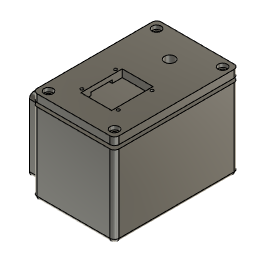
memento-mori (Autodesk Fusion 360 design; units mm, degrees)
Autodesk Fusion 360 part; units mm, degrees
sketch "pcb" plane through (0, 0, 0) normal (0, 0, 1) x (1, 0, 0)
  line L0 (0, 0) -> (40, 0)
  line L1 (40, 0) -> (40, 60.5)
  line L2 (40, 60.5) -> (0, 60.5)
  line L3 (0, 60.5) -> (0, 0)
  line L4 (2.25, 60.5) -> (2.25, 67.8)
  line L5 (2.25, 67.8) -> (21.25, 67.8)
  line L6 (21.25, 67.8) -> (21.25, 60.5)
  circle A0 centre (37.1, 57.8) radius 0.9
  line L7 (20, 0) -> (20, 60.5) construction
  line L8 (0, 30.25) -> (40, 30.25) construction
  circle A1 centre (2.9, 57.8) radius 0.9
  circle A2 centre (2.9, 2.7) radius 0.9
  circle A3 centre (37.1, 2.7) radius 0.9
  dimension "d1" = 40
  dimension "d2" = 60.5
  dimension "d5" = 2.25
  dimension "d6" = 19
  dimension "d7" = 7.3
  dimension "d12" = 1.8
  dimension "d13" = 1.8
  dimension "d14" = 2
  constraint horizontal L0
  constraint vertical L1
  constraint horizontal L2
  constraint vertical L3
  constraint coincident L0.start L3.end
  constraint coincident L2 L4.start
  constraint perpendicular L2 L4
  constraint perpendicular L4 L5
  constraint coincident L2 L6.end
  constraint perpendicular L2 L6
  constraint midpoint L0 L7.start
  constraint midpoint L2 L7.end
  constraint midpoint L3 L8.start
  constraint midpoint L1 L8.end
  constraint symmetric A0 L7 A1
  constraint symmetric A0 L8 A3
  constraint symmetric L8 A1 A2
  measures "d1" distance of L0.start L0.end
  measures "d2" distance of L0.start L2.end
  measures "d5" distance of L3 L4
  measures "d6" distance of L4.end L5.end
  measures "d7" distance of L5.end L6.end
  measures "d12" diameter of A0
  measures "d13" distance of L2 A0
  measures "d14" distance of L1 A0
extrude "Extrude1" add sketch "pcb" along normal blind 20 makes body 1
sketch "case" plane through (0, 0, 20) normal (0, 0, 1) x (-1, 0, 0)
  line L0 (-2.25, -60.5) -> (0, -60.5)
  line L1 (0, -60.5) -> (0, 0)
  line L2 (0, 0) -> (-40, 0)
  line L3 (-40, 0) -> (-40, -60.5)
  line L4 (-40, -60.5) -> (-21.25, -60.5)
  line L5 (-21.25, -60.5) -> (-21.25, -67.8)
  line L6 (-21.25, -67.8) -> (-2.25, -67.8)
  line L7 (-2.25, -67.8) -> (-2.25, -60.5)
  line L8 (7, -69.8) -> (-47, -69.8)
  line L9 (-47, -69.8) -> (-47, 12)
  line L10 (-47, 12) -> (7, 12)
  line L11 (7, 12) -> (7, -69.8)
  line L12 (-40, 0) -> (-40, -60.5)
  line L13 (0, -60.5) -> (0, 0)
  line L14 (0, 0) -> (-40, 0)
  line L15 (-2.25, -67.8) -> (-21.25, -67.8)
  circle A0 centre (-37.1, -2.7) radius 0.9
  circle A1 centre (-2.9, -2.7) radius 0.9
  circle A2 centre (-2.9, -57.8) radius 0.9
  circle A3 centre (-37.1, -57.8) radius 0.9
  line L16 (-44.25, 9.25) -> (4.25, 9.25)
  line L17 (4.25, 9.25) -> (4.25, -67.05)
  line L18 (4.25, -67.05) -> (-44.25, -67.05)
  line L19 (-44.25, -67.05) -> (-44.25, 9.25)
  dimension "d8" = 7
  dimension "d9" = 7
  dimension "d10" = 12
  dimension "d11" = 2
  dimension "d15" = 2.75
  constraint horizontal L8
  constraint vertical L9
  constraint horizontal L10
  constraint vertical L11
  measures "d8" distance of L9 L12
  measures "d9" distance of L11 L13
  measures "d10" distance of L10 L14
  measures "d11" distance of L8 L15
extrude "Extrude3" add sketch "case" against normal blind 8.5 from surface at -20 separate body contours L0 L1 L2 L3 L4 L5 L7 L12 L13 L14 L18 | L0 L1 L2 L3 L4 L5 L7 L12 L13 L14 L16 L17 L18 L19 | L5 L6 L7 L15 L18 | L8 L9 L10 L11 | A0 | A1 | A2 | A3 makes body 2
extrude "Extrude4" add sketch "case" along normal blind 45 from surface at -20 contours L5 L6 L7 L15 L18 | L8 L9 L10 L11 bodies 2
sketch "charge-panel" plane through (0, 69.8, 0) normal (0, 1, 0) x (-1, 0, 0)
  line L0 (-47, 45) -> (-47, -8.5)
  line L1 (-47, -8.5) -> (7, -8.5)
  line L2 (7, -8.5) -> (7, 45)
  line L3 (7, 45) -> (-47, 45)
  line L4 (-21.25, 0) -> (-21.25, 20)
  line L5 (-21.25, 20) -> (-2.25, 20) construction
  line L6 (-2.25, 0) -> (-2.25, 20)
  line L7 (-2.25, 0) -> (-21.25, 0)
  line L8 (-40, 20) -> (-21.25, 20)
  line L9 (-40, 0) -> (-40, 20)
  line L10 (-40, 0) -> (-21.25, 0)
  line L11 (0, 0) -> (0, 20)
  line L12 (-2.25, 0) -> (0, 0)
  line L13 (-2.25, 20) -> (0, 20)
  line L14 (-21.25, 25) -> (-2.25, 25)
  line L15 (-21.25, 25) -> (-26, 25)
  line L16 (-26, 25) -> (-26, 0)
  line L17 (-38, 25) -> (-34, 25)
  line L18 (-34, 25) -> (-34, 16.35)
  line L19 (-34, 16.35) -> (-38, 16.35)
  line L20 (-38, 16.35) -> (-38, 25)
  line L21 (-21.25, 10) -> (-2.25, 10)
  line L22 (-21.25, 20) -> (-21.25, 25)
  line L23 (-2.25, 25) -> (-2.25, 20)
  dimension "d28" = 4.75
  dimension "d29" = 8.65
  dimension "d30" = 4
  dimension "d32" = 2
  dimension "d160" = 10
  dimension "d161" = 15
  constraint coincident L4 L14.start
  constraint coincident L6 L14.end
  constraint perpendicular L6 L14
  constraint perpendicular L4 L15
  constraint coincident L10 L16.end
  constraint horizontal L17
  constraint vertical L18
  constraint horizontal L19
  constraint vertical L20
  constraint coincident L4 L21.start
  constraint coincident L6 L21.end
  constraint perpendicular L6 L21
  constraint coincident L4.end L5.start
  constraint coincident L5.end L6.end
  constraint collinear L15 L17
  measures "d28" distance of L4 L16
  measures "d29" distance of L17.end L18.end
  measures "d30" distance of L17.start L17.end
  measures "d32" distance of L9 L20
  measures "d160" distance of L7 L21
  measures "d161" distance of L14 L21
extrude "Extrude5" cut sketch "charge-panel" against normal up to surface (2.75 mm away) contours L8 L18 L19 L20 | L8 L17 L18 L20 bodies 2
extrude "Extrude6" cut sketch "charge-panel" against normal up to surface (2.75 mm away) contours L4 L6 L14 L21 L22 L23 bodies 1 2
fillet "Fillet2" radius 3 4 edges at (-7, -12, 18.25) (47, -12, 18.25) (47, 69.8, 18.25) (-7, 69.8, 18.25) on bodies 2
sketch "holes" plane through (0, 0, 45) normal (0, 0, 1) x (-1, 0, 0)
  line L0 (-44.25, -67.05) -> (-44.25, 9.25)
  line L1 (-44.25, 9.25) -> (4.25, 9.25)
  line L2 (4.25, 9.25) -> (4.25, -67.05)
  line L3 (4.25, -67.05) -> (-44.25, -67.05)
  arc A0 (4, -69.8) -> (7, -66.8) centre (4, -66.8) ccw
  line L4 (7, -66.8) -> (7, 9)
  arc A1 (7, 9) -> (4, 12) centre (4, 9) ccw
  line L5 (4, 12) -> (-44, 12)
  arc A2 (-44, 12) -> (-47, 9) centre (-44, 9) ccw
  line L6 (-47, 9) -> (-47, -66.8)
  arc A3 (-47, -66.8) -> (-44, -69.8) centre (-44, -66.8) ccw
  line L7 (-44, -69.8) -> (4, -69.8)
  line L8 (4.25, 9.25) -> (4.25, -67.05)
  line L9 (4.25, -67.05) -> (-44.25, -67.05)
  line L10 (-44.25, -67.05) -> (-44.25, 9.25)
  line L11 (-44.25, 9.25) -> (4.25, 9.25)
  line L12 (4.25, -61.948) -> (-0.75, -61.948)
  line L13 (-0.75, -61.948) -> (-0.75, -67.05)
  line L14 (-20, -67.05) -> (-20, 9.25) construction
  line L15 (4.25, -28.9) -> (-44.25, -28.9) construction
  line L16 (1.75, -61.948) -> (1.75, -67.05) construction
  line L17 (-0.75, -64.499) -> (4.25, -64.499) construction
  circle A4 centre (1.75, -64.499) radius 1.425
  circle A5 centre (1.75, -64.499) radius 2.95
  circle A6 centre (-41.75, -64.499) radius 1.425
  circle A7 centre (-41.75, -64.499) radius 2.95
  line L18 (-44.25, -61.948) -> (-39.25, -61.948)
  line L19 (-39.25, -61.948) -> (-39.25, -67.05)
  circle A8 centre (1.75, 6.699) radius 2.95
  circle A9 centre (1.75, 6.699) radius 1.425
  line L20 (-0.75, 4.148) -> (-0.75, 9.25)
  line L21 (4.25, 4.148) -> (-0.75, 4.148)
  line L22 (-44.25, 4.148) -> (-39.25, 4.148)
  line L23 (-39.25, 4.148) -> (-39.25, 9.25)
  circle A10 centre (-41.75, 6.699) radius 2.95
  circle A11 centre (-41.75, 6.699) radius 1.425
  circle A12 centre (-41.75, -64.499) radius 1.675
  circle A13 centre (1.75, -64.499) radius 1.675
  circle A14 centre (-41.75, 6.699) radius 1.675
  circle A15 centre (1.75, 6.699) radius 1.675
  dimension "d50" = 5
  dimension "d51" = 5.102
  dimension "d53" = 2.85
  dimension "d54" = 5.9
  dimension "d66" = 0.25
  constraint coincident L8 L12.start
  constraint perpendicular L8 L12
  constraint coincident L9 L13.end
  constraint perpendicular L9 L13
  constraint midpoint L9 L14.start
  constraint midpoint L11 L14.end
  constraint midpoint L8 L15.start
  constraint midpoint L10 L15.end
  constraint midpoint L12 L16.start
  constraint coincident L9 L16.end
  constraint perpendicular L9 L16
  constraint midpoint L13 L17.start
  constraint coincident L8 L17.end
  constraint perpendicular L8 L17
  constraint midpoint L17 A4.centre
  constraint concentric A4 A5
  constraint symmetric L12.start L14 L18.start
  constraint symmetric L12.end L14 L18.end
  constraint symmetric L13.end L14 L19.end
  constraint symmetric L14 A4 A6
  constraint symmetric L14 A5 A7
  constraint symmetric L12.start L15 L21.start
  constraint symmetric L12.end L15 L20.start
  constraint symmetric L13.end L15 L20.end
  constraint symmetric L15 A4 A9
  constraint symmetric L15 A5 A8
  constraint symmetric L15 A6 A11
  constraint symmetric L15 A7 A10
  constraint symmetric L15 L18.start L22.start
  constraint symmetric L15 L18.end L22.end
  constraint symmetric L15 L19.end L23.end
  constraint symmetric L14 A12 A13
  constraint symmetric L15 A12 A14
  constraint symmetric L15 A13 A15
  measures "d50" distance of L12.start L12.end
  measures "d51" distance of L12.end L13.end
  measures "d53" diameter of A4
  measures "d54" diameter of A5
extrude "Extrude8" add sketch "holes" against normal up to surface (45 mm away) contours L0 L10 A7 L18 | L0 L10 L22 A10 | L0 L3 L9 L10 A7 L18 L19 | L0 L1 L10 L11 L22 L23 A10 | L0 L3 L9 L10 A7 | A7 L18 L19 | L0 L1 L10 L11 A10 | L22 L23 A10 | L3 L9 A7 L19 | L1 L11 L23 A10 | L3 L9 L13 A5 | L1 L11 A8 L20 | L2 L3 L8 L9 L12 L13 A5 | L1 L2 L8 L11 A8 L20 L21 | L2 L3 L8 L9 A5 | L12 L13 A5 | L1 L2 L8 L11 A8 | A8 L20 L21 | L2 L8 L12 A5 | L2 L8 A8 L21 | A4 | A6 | A9 | A11 | A12 | A13 | A14 | A15 bodies 2
extrude "Extrude9" cut sketch "holes" against normal blind 8 contours A4 | A6 | A9 | A11 bodies 2
fillet "Fillet3" radius 2 4 edges at (0.75, 61.948, 22.5) (39.25, 61.948, 22.5) (0.75, -4.148, 22.5) (39.25, -4.148, 22.5) on bodies 2
extrude "Extrude10" add sketch "case" along normal blind 5 from surface at 25 separate body contours L0 L1 L2 L3 L4 L5 L7 L12 L13 L14 L18 | L0 L1 L2 L3 L4 L5 L7 L12 L13 L14 L16 L17 L18 L19 | L5 L6 L7 L15 L18 | L8 L9 L10 L11 | A0 | A1 | A2 | A3 makes body 3
fillet "Fillet4" radius 3 4 edges at (47, 69.8, 47.5) (-7, 69.8, 47.5) (-7, -12, 47.5) (47, -12, 47.5) on bodies 3
extrude "Extrude11" cut sketch "holes" along normal up to surface (5 mm away) contours A4 | A6 | A9 | A11 | A12 | A13 | A14 | A15 bodies 3
extrude "Extrude12" cut sketch "holes" against normal blind 2.5 from surface at 5 contours L0 L3 L9 L10 A7 L18 L19 | L0 L10 A7 | A7 L18 | L0 L10 A10 | L0 L1 L10 L11 L22 L23 A10 | L22 A10 | L3 L9 A7 | A7 L19 | L1 L11 A10 | L23 A10 | L2 L3 L8 L9 L12 L13 A5 | L3 L9 A5 | L13 A5 | L1 L11 A8 | L1 L2 L8 L11 A8 L20 L21 | A8 L20 | L2 L8 A5 | L12 A5 | L2 L8 A8 | A8 L21 bodies 3
move_body "Move1" bodies 3 to x (1, 0, 0) y (0, 1, 0) z (0, 0, 1) at (0, 0, 2.5)
sketch "lid-holes" plane through (0, 0, 52.5) normal (0, 0, 1) x (-1, 0, 0)
  circle A0 centre (-41.75, -64.499) radius 2.95
  circle A1 centre (-41.75, 6.699) radius 2.95
  circle A2 centre (1.75, -64.499) radius 2.95
  circle A3 centre (1.75, 6.699) radius 2.95
  arc A4 (-44, 12) -> (-47, 9) centre (-44, 9) ccw
  line L0 (-47, 9) -> (-47, -66.8)
  arc A5 (-47, -66.8) -> (-44, -69.8) centre (-44, -66.8) ccw
  line L1 (-44, -69.8) -> (4, -69.8)
  arc A6 (4, -69.8) -> (7, -66.8) centre (4, -66.8) ccw
  line L2 (7, -66.8) -> (7, 9)
  arc A7 (7, 9) -> (4, 12) centre (4, 9) ccw
  line L3 (4, 12) -> (-44, 12)
  line L4 (4, 12) -> (-44, 12)
  arc A8 (7, 9) -> (4, 12) centre (4, 9) ccw
  line L5 (7, -66.8) -> (7, 9)
  line L6 (-47, 9) -> (-47, -66.8)
  arc A9 (-44, 12) -> (-47, 9) centre (-44, 9) ccw
  arc A10 (-47, -66.8) -> (-44, -69.8) centre (-44, -66.8) ccw
  line L7 (-44, -69.8) -> (4, -69.8)
  arc A11 (4, -69.8) -> (7, -66.8) centre (4, -66.8) ccw
  circle A12 centre (1.75, -64.499) radius 2.95
  circle A13 centre (1.75, 6.699) radius 2.95
  circle A14 centre (-41.75, 6.699) radius 2.95
  circle A15 centre (-41.75, -64.499) radius 2.95
  line L8 (-20, 12) -> (-20, -69.8) construction
  line L9 (-9.875, -3) -> (-30.125, -3)
  line L10 (-30.125, -3) -> (-30.125, -30.25)
  line L11 (-30.125, -30.25) -> (-9.875, -30.25)
  line L12 (-9.875, -30.25) -> (-9.875, -3)
  line L13 (-6.375, -2.25) -> (-33.625, -2.25)
  line L14 (-33.625, -2.25) -> (-33.625, -31)
  line L15 (-33.625, -31) -> (-6.375, -31)
  line L16 (-6.375, -31) -> (-6.375, -2.25)
  line L17 (-6.375, -16.625) -> (-33.625, -16.625) construction
  line L18 (-20, -2.25) -> (-20, -31) construction
  line L19 (-9.875, -16.625) -> (-30.125, -16.625) construction
  circle A16 centre (-7.375, -3.25) radius 1
  circle A17 centre (-7.375, -30) radius 1
  circle A18 centre (-32.625, -3.25) radius 1
  circle A19 centre (-32.625, -30) radius 1
  circle A20 centre (-7.375, -3.25) radius 1.9
  circle A21 centre (-7.375, -30) radius 1.9
  circle A22 centre (-32.625, -3.25) radius 1.9
  circle A23 centre (-32.625, -30) radius 1.9
  circle A24 centre (-20, -51.35) radius 3.45
  line L20 (-35.625, -0.25) -> (-35.625, -33)
  line L21 (-35.625, -33) -> (-4.375, -33)
  line L22 (-4.375, -33) -> (-4.375, -0.25)
  line L23 (-4.375, -0.25) -> (-35.625, -0.25)
  point P0 (-20, -3)
  point P1 (-20, -16.625)
  point P2 (-20, -16.625)
  dimension "d72" = 20.25
  dimension "d73" = 27.25
  dimension "d74" = 15
  dimension "d75" = 27.25
  dimension "d76" = 28.75
  dimension "d77" = 2
  dimension "d78" = 3.8
  dimension "d79" = 6.9
  dimension "d80" = 15
  dimension "d87" = 2
  constraint midpoint L3 L8.start
  constraint midpoint L7 L8.end
  constraint horizontal L9
  constraint vertical L10
  constraint horizontal L11
  constraint vertical L12
  constraint midpoint L9 P0
  constraint coincident L8 P0
  constraint horizontal L13
  constraint vertical L14
  constraint horizontal L15
  constraint vertical L16
  constraint midpoint L16 L17.start
  constraint midpoint L14 L17.end
  constraint midpoint L13 L18.start
  constraint midpoint L15 L18.end
  constraint midpoint L18 P2
  constraint midpoint L12 L19.start
  constraint midpoint L10 L19.end
  constraint midpoint L19 P2
  constraint coincident P2 P1
  constraint tangent L16 A16
  constraint tangent L13 A16
  constraint symmetric L17 A16 A17
  constraint symmetric L8 A16 A18
  constraint symmetric L8 A17 A19
  constraint concentric A16 A20
  constraint symmetric L17 A20 A21
  constraint symmetric L8 A20 A22
  constraint symmetric L8 A21 A23
  constraint coincident L8 A24.centre
  measures "d72" distance of L9.start L9.end
  measures "d73" distance of L9.start L11.end
  measures "d74" distance of L4 L9
  measures "d75" distance of L13.start L13.end
  measures "d76" distance of L13.start L15.end
  measures "d77" diameter of A16
  measures "d78" diameter of A20
  measures "d79" diameter of A24
  measures "d80" distance of L1 A24
extrude "Extrude15" cut sketch "lid-holes" against normal blind 5 contours L9 L10 L11 L12 bodies 3
sketch "lid-offset" plane through (0, 0, 47.5) normal (0, 0, -1) x (1, 0, 0)
  circle A0 centre (-1.75, 6.699) radius 1.675
  circle A1 centre (41.75, -64.499) radius 1.675
  circle A2 centre (41.75, 6.699) radius 1.675
  circle A3 centre (-1.75, -64.499) radius 1.675
  arc A4 (47, 9) -> (44, 12) centre (44, 9) ccw
  line L0 (44, 12) -> (-4, 12)
  arc A5 (-4, 12) -> (-7, 9) centre (-4, 9) ccw
  line L1 (-7, 9) -> (-7, -66.8)
  arc A6 (-7, -66.8) -> (-4, -69.8) centre (-4, -66.8) ccw
  line L2 (-4, -69.8) -> (44, -69.8)
  arc A7 (44, -69.8) -> (47, -66.8) centre (44, -66.8) ccw
  line L3 (47, -66.8) -> (47, 9)
  line L4 (-2, 2.524) -> (42, 2.524)
  line L5 (42, 2.524) -> (42, -60.324)
  line L6 (42, -60.324) -> (-2, -60.324)
  line L7 (-2, -60.324) -> (-2, 2.524)
  line L8 (9.875, -30.25) -> (30.125, -30.25)
  line L9 (30.125, -30.25) -> (30.125, -3)
  line L10 (30.125, -3) -> (9.875, -3)
  line L11 (9.875, -3) -> (9.875, -30.25)
  line L12 (9.875, -3) -> (30.125, -3)
  line L13 (30.125, -3) -> (30.125, -30.25)
  line L14 (30.125, -30.25) -> (9.875, -30.25)
  line L15 (9.875, -30.25) -> (9.875, -3)
  line L16 (9.875, -16.625) -> (-2, -16.625) construction
  line L17 (1.875, -9.625) -> (9.875, -9.625)
  line L18 (9.875, -9.625) -> (9.875, -23.625)
  line L19 (9.875, -23.625) -> (1.875, -23.625)
  line L20 (1.875, -23.625) -> (1.875, -9.625)
  line L21 (1.875, -16.625) -> (9.875, -16.625) construction
  line L22 (5.875, -9.625) -> (5.875, -23.625) construction
  line L23 (20, -3) -> (20, -30.25) construction
  line L24 (38.125, -9.625) -> (30.125, -9.625)
  line L25 (38.125, -23.625) -> (38.125, -9.625)
  line L26 (30.125, -23.625) -> (38.125, -23.625)
  point P0 (5.875, -16.625)
  dimension "d109" = 5
  dimension "d111" = 5
  dimension "d112" = 2.5
  dimension "d113" = 2.5
  dimension "d147" = 8
  dimension "d148" = 14
  constraint horizontal L4
  constraint vertical L5
  constraint horizontal L6
  constraint vertical L7
  constraint midpoint L15 L16.start
  constraint coincident L7 L16.end
  constraint perpendicular L7 L16
  constraint horizontal L17
  constraint vertical L18
  constraint horizontal L19
  constraint vertical L20
  constraint midpoint L20 L21.start
  constraint midpoint L18 L16.start
  constraint midpoint L17 L22.start
  constraint midpoint L19 L22.end
  constraint midpoint L22 P0
  constraint coincident L16 P0
  constraint coincident L16.start L18
  constraint midpoint L10 L23.start
  constraint midpoint L14 L23.end
  constraint symmetric L17.start L23 L24.start
  constraint symmetric L17.end L23 L24.end
  constraint symmetric L18.end L23 L26.start
  constraint symmetric L19.end L23 L25.start
  measures "d109" distance of L3 L5
  measures "d111" distance of L1 L7
  measures "d112" distance of A0 L4
  measures "d113" distance of A3 L6
  measures "d147" distance of L17.start L17.end
  measures "d148" distance of L17.start L19.end
extrude "Extrude23" cut sketch "lid-offset" along normal blind 7 from surface at -1 contours L4 L5 L6 L7 | L8 L9 L10 L11 L12 L13 L14 L15 L18 | L11 L15 L17 L18 L19 L20 | L9 L13 L24 L25 L26 bodies 3
extrude "Extrude24" cut sketch "lid-holes" against normal up to surface (4 mm away) contours A24 bodies 3
sketch "feet" plane through (-7, 0, 0) normal (-1, 0, 0) x (0, -1, 0)
  line L0 (-66.8, 45) -> (-66.8, -8.5)
  line L1 (-66.8, -8.5) -> (9, -8.5)
  line L2 (9, -8.5) -> (9, 45)
  line L3 (9, 45) -> (-66.8, 45)
  line L4 (-66.8, 45) -> (9, 45)
  line L5 (-66.8, -8.5) -> (-66.8, 45)
  line L6 (9, -8.5) -> (-66.8, -8.5)
  line L7 (9, 45) -> (9, -8.5)
  line L8 (-28.9, 45) -> (-28.9, -8.5) construction
  line L9 (-66.8, 18.25) -> (9, 18.25) construction
  line L10 (-61.8, 42) -> (-51.8, 42)
  line L11 (-51.8, 42) -> (-51.8, -5.5)
  line L12 (-51.8, -5.5) -> (-61.8, -5.5)
  line L13 (-61.8, -5.5) -> (-61.8, 42)
  line L14 (4, 42) -> (-6, 42)
  line L15 (4, -5.5) -> (4, 42)
  line L16 (-6, 42) -> (-6, -5.5)
  line L17 (-6, -5.5) -> (4, -5.5)
  dimension "d125" = 3
  dimension "d126" = 5
  dimension "d131" = 3
  dimension "d132" = 10
  constraint midpoint L4 L8.start
  constraint midpoint L6 L8.end
  constraint midpoint L5 L9.start
  constraint midpoint L7 L9.end
  constraint horizontal L10
  constraint vertical L11
  constraint horizontal L12
  constraint vertical L13
  constraint symmetric L8 L10.start L14.start
  constraint symmetric L8 L10.end L14.end
  constraint symmetric L8 L11.end L16.end
  constraint symmetric L8 L12.end L15.start
  measures "d125" distance of L3 L10
  measures "d126" distance of L0 L13
  measures "d131" distance of L1 L12
  measures "d132" distance of L10.start L10.end
extrude "Extrude26" add sketch "feet" along normal blind 10 contours L10 L11 L12 L13 | L14 L15 L16 L17 bodies 2
fillet "Fillet8" radius 3 8 edges at (-12, 61.8, 42) (-12, 51.8, 42) (-12, 6, 42) (-12, -4, 42) (-12, -4, -5.5) (-12, 6, -5.5) (-12, 51.8, -5.5) (-12, 61.8, -5.5) on bodies 2
sketch "pcb-mount" plane through (0, 0, 0) normal (0, 0, 1) x (-1, 0, 0)
  line L0 (-39.25, -67.05) -> (-0.75, -67.05)
  line L1 (-0.75, -67.05) -> (-0.75, -63.948)
  arc A0 (1.25, -61.948) -> (-0.75, -63.948) centre (1.25, -63.948) ccw
  line L2 (1.25, -61.948) -> (4.25, -61.948)
  line L3 (4.25, -61.948) -> (4.25, 4.148)
  line L4 (4.25, 4.148) -> (1.25, 4.148)
  arc A1 (-0.75, 6.148) -> (1.25, 4.148) centre (1.25, 6.148) ccw
  line L5 (-0.75, 6.148) -> (-0.75, 9.25)
  line L6 (-0.75, 9.25) -> (-39.25, 9.25)
  line L7 (-39.25, 9.25) -> (-39.25, 6.148)
  arc A2 (-41.25, 4.148) -> (-39.25, 6.148) centre (-41.25, 6.148) ccw
  line L8 (-41.25, 4.148) -> (-44.25, 4.148)
  line L9 (-44.25, 4.148) -> (-44.25, -61.948)
  line L10 (-44.25, -61.948) -> (-41.25, -61.948)
  arc A3 (-39.25, -63.948) -> (-41.25, -61.948) centre (-41.25, -63.948) ccw
  line L11 (-39.25, -63.948) -> (-39.25, -67.05)
  circle A4 centre (-37.1, -57.8) radius 0.9
  circle A5 centre (-2.9, -57.8) radius 0.9
  circle A6 centre (-37.1, -2.7) radius 0.9
  circle A7 centre (-2.9, -2.7) radius 0.9
  circle A8 centre (-37.1, -2.7) radius 1.225
  line L12 (-20, 9.25) -> (-20, -67) construction
  line L13 (-44.25, -28.9) -> (4.25, -28.9) construction
  circle A9 centre (-2.9, -2.7) radius 1.225
  circle A10 centre (-37.1, -57.8) radius 1.225
  circle A11 centre (-2.9, -57.8) radius 1.225
  dimension "d139" = 2.45
  dimension "d140" = 2.45
  constraint concentric A6 A8
  constraint midpoint L6 L12.start
  constraint perpendicular L6 L12
  constraint midpoint L9 L13.start
  constraint midpoint L3 L13.end
  constraint symmetric A8 L12 A9
  constraint concentric A4 A10
  constraint symmetric L12 A10 A11
  measures "d139" diameter of A8
  measures "d140" diameter of A10
extrude "Extrude27" cut sketch "pcb-mount" against normal blind 6 contours A4 | A5 | A6 | A7 | A8 | A9 | A10 | A11 bodies 2
fillet "Fillet10" radius 3 4 edges at (-2, 60.324, 48) (-2, -2.524, 48) (42, -2.524, 48) (42, 60.324, 48) on bodies 3
fillet "Fillet11" radius 2.5 8 edges at (46.1213, -11.1213, -8.5) (20, -12, -8.5) (-6.1213, -11.1213, -8.5) (-7, 28.9, -8.5) (-6.1213, 68.9213, -8.5) (20, 69.8, -8.5) (46.1213, 68.9213, -8.5) (47, 28.9, -8.5) on bodies 2
extrude "Extrude28" cut sketch "lid-offset" against normal blind 2 contours L11 L15 L17 L18 L19 L20 | L9 L13 L24 L25 L26 bodies 3
extrude "Extrude29" add 1 faces at (31.7444, 45.809, 48.5) along direction (0, 0, -1) up to surface (1 mm away) on bodies 3 bodies 3
sketch "display-mount" plane through (0, 0, 52.5) normal (0, 0, 1) x (-1, 0, 0)
  circle A0 centre (-20, -51.35) radius 3.45
  line L0 (-30.125, -3) -> (-9.875, -3)
  line L1 (-9.875, -3) -> (-9.875, -30.25)
  line L2 (-9.875, -30.25) -> (-30.125, -30.25)
  line L3 (-30.125, -30.25) -> (-30.125, -3)
  circle A1 centre (-41.75, -64.499) radius 2.95
  circle A2 centre (-41.75, 6.699) radius 2.95
  circle A3 centre (1.75, -64.499) radius 2.95
  circle A4 centre (1.75, 6.699) radius 2.95
  arc A5 (-44, 12) -> (-47, 9) centre (-44, 9) ccw
  line L4 (-47, 9) -> (-47, -66.8)
  arc A6 (-47, -66.8) -> (-44, -69.8) centre (-44, -66.8) ccw
  line L5 (-44, -69.8) -> (4, -69.8)
  arc A7 (4, -69.8) -> (7, -66.8) centre (4, -66.8) ccw
  line L6 (7, -66.8) -> (7, 9)
  arc A8 (7, 9) -> (4, 12) centre (4, 9) ccw
  line L7 (4, 12) -> (-44, 12)
  circle A9 centre (-32.025, -27.75) radius 0.95
  circle A10 centre (-32.025, -27.75) radius 1.9
  line L8 (-9.875, -16.625) -> (-30.125, -16.625) construction
  line L9 (-20, -3) -> (-20, -30.25) construction
  line L10 (-30.125, -30.25) -> (-37.506, -30.25) construction
  circle A11 centre (-32.025, -5.5) radius 1.9
  circle A12 centre (-32.025, -5.5) radius 0.95
  circle A13 centre (-7.975, -27.75) radius 1.9
  circle A14 centre (-7.975, -27.75) radius 0.95
  circle A15 centre (-7.975, -5.5) radius 1.9
  circle A16 centre (-7.975, -5.5) radius 0.95
  dimension "d153" = 1.9
  dimension "d154" = 3.8
  dimension "d159" = 2.5
  constraint concentric A9 A10
  constraint midpoint L1 L8.start
  constraint midpoint L3 L8.end
  constraint midpoint L0 L9.start
  constraint midpoint L2 L9.end
  constraint tangent L3 A10
  constraint coincident L2.end L3.start
  constraint perpendicular L3 L10
  constraint symmetric A9 L8 A12
  constraint symmetric A10 L8 A11
  constraint symmetric A9 L9 A14
  constraint symmetric A10 L9 A13
  constraint symmetric L9 A11 A15
  constraint symmetric L9 A12 A16
  measures "d153" diameter of A9
  measures "d154" diameter of A10
  measures "d159" distance of A9.centre L10
extrude "Extrude31" cut sketch "display-mount" against normal up to surface (5 mm away) contours A9 | A12 | A14 | A16 bodies 3
fillet "Fillet12" radius 1.5 4 edges at (21.25, 68.425, 25) (2.25, 68.425, 25) (2.25, 68.425, 10) (21.25, 68.425, 10) on bodies 2
hidden bodies 1
named bodies: "pcb", "case", "lid"
